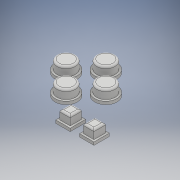
# Autodesk Inventor part: Groboy Buttons
Saved by Autodesk Inventor 2017 SP1 (Build 210196100, 196)
## iProperties
Created: 2017-10-10
Part Number: Groboy Buttons
Material: Generic
Document SubType Name: Modeling
Designer: Groguard
Density: 1 g/cm^3
Appearance: Default
Author: Groguard
Autodesk Inventor part; units mm, degrees
ref_plane "YZ Plane" through (0, 0, 0) normal (1, 0, 0) x (0, 1, 0)
ref_plane "XZ Plane" through (0, 0, 0) normal (0, 1, 0) x (-1, 0, 0)
ref_plane "XY Plane" through (0, 0, 0) normal (0, 0, 1) x (1, 0, 0)
sketch "Sketch1" plane through (0, 0, 0) normal (0, 0, 1) x (1, 0, 0)
  circle A0 centre (22, 46) radius 4.5
  circle A1 centre (12, 36) radius 4.5
  circle A2 centre (22, 26) radius 4.5
  circle A3 centre (32, 36) radius 4.5
  line L0 (37.75, 18) -> (32.5, 18)
  line L1 (32.5, 18) -> (32.5, 12.25)
  line L2 (32.5, 12.25) -> (37.75, 12.25)
  line L3 (37.75, 12.25) -> (37.75, 18)
  line L4 (44.5, 18) -> (49.75, 18)
  line L5 (49.75, 18) -> (49.75, 12.25)
  line L6 (49.75, 12.25) -> (44.5, 12.25)
  line L7 (44.5, 12.25) -> (44.5, 18)
  circle A4 centre (12, 36) radius 5.625
  circle A5 centre (22, 46) radius 5.625
  circle A6 centre (32, 36) radius 5.625
  circle A7 centre (22, 26) radius 5.625
  line L8 (38.75, 19) -> (31.5, 19)
  line L9 (31.5, 19) -> (31.5, 11.25)
  line L10 (31.5, 11.25) -> (38.75, 11.25)
  line L11 (38.75, 11.25) -> (38.75, 19)
  line L12 (50.75, 19) -> (43.5, 19)
  line L13 (43.5, 19) -> (43.5, 11.25)
  line L14 (43.5, 11.25) -> (50.75, 11.25)
  line L15 (50.75, 11.25) -> (50.75, 19)
  point P0 (18.75, 39)
  point P1 (18.75, 32.5)
  dimension "d35" = 11.25
  dimension "d36" = 11.25
  dimension "d37" = 11.25
  dimension "d38" = 11.25
  dimension "d43" = 7.75
  dimension "d44" = 7.75
  dimension "d45" = 7.25
  dimension "d46" = 7.25
  dimension "d47" = 5.75
  dimension "d48" = 5.25
  dimension "d49" = 5.75
  dimension "d50" = 5.25
  constraints: 32 end point, 8 centre point, 8 parallel, 4 perpendicular
  measures "d35" diameter of A4
  measures "d36" diameter of A7
  measures "d37" diameter of A6
  measures "d38" diameter of A5
  measures "d43" distance between parallel lines of L10 L8
  measures "d44" distance between parallel lines of L14 L12
  measures "d45" distance between parallel lines of L11 L9
  measures "d46" distance between parallel lines of L15 L13
  measures "d47" distance between parallel lines of L6 L4
  measures "d48" distance between parallel lines of L7 L5
  measures "d49" distance between parallel lines of L2 L0
  measures "d50" distance between parallel lines of L1 L3
extrude "Extrusion1" add sketch "Sketch1" along normal blind 6 contours A0 | A1 | A2 | A3 | L3 L2 L1 L0 | L4 L5 L6 L7 | A4 | A5 | A6 | A7 | L11 L10 L9 L8 | L15 L14 L13 L12
sketch "Sketch2" plane through (0, 0, 6) normal (0, 0, 1) x (1, 0, 0)
  circle A0 centre (22, 46) radius 4.625
  circle A1 centre (12, 36) radius 4.625
  circle A2 centre (22, 26) radius 4.625
  circle A3 centre (32, 36) radius 4.625
  circle A4 centre (22, 46) radius 5.625
  circle A5 centre (12, 36) radius 5.625
  circle A6 centre (22, 26) radius 5.625
  circle A7 centre (32, 36) radius 5.625
  line L0 (31.5, 19) -> (31.5, 11.25) projected
  line L1 (38.75, 11.25) -> (38.75, 19) projected
  line L2 (31.5, 19) -> (38.75, 19)
  line L3 (38.75, 19) -> (38.75, 11.25)
  line L4 (38.75, 11.25) -> (31.5, 11.25)
  line L5 (31.5, 11.25) -> (31.5, 19)
  line L6 (50.75, 19) -> (43.5, 19) projected
  line L7 (43.5, 11.25) -> (50.75, 11.25) projected
  line L8 (43.5, 19) -> (50.75, 19)
  line L9 (50.75, 19) -> (50.75, 11.25)
  line L10 (50.75, 11.25) -> (43.5, 11.25)
  line L11 (43.5, 11.25) -> (43.5, 19)
  line L12 (37.75, 18) -> (32.5, 18)
  line L13 (32.5, 18) -> (32.5, 12.25)
  line L14 (32.5, 12.25) -> (37.75, 12.25)
  line L15 (37.75, 12.25) -> (37.75, 18)
  line L16 (44.5, 18) -> (49.75, 18)
  line L17 (49.75, 18) -> (49.75, 12.25)
  line L18 (49.75, 12.25) -> (44.5, 12.25)
  line L19 (44.5, 12.25) -> (44.5, 18)
  dimension "d16" = 1
  dimension "d17" = 1
  dimension "d18" = 1
  dimension "d19" = 1
  dimension "d39" = 11.25
  dimension "d40" = 11.25
  dimension "d41" = 11.25
  dimension "d42" = 11.25
  dimension "d51" = 1
  dimension "d52" = 1
  constraints: 32 end point, 8 centre point, 8 parallel, 4 perpendicular, 2 horizontal, 6 other
  measures "d16" radial gap between concentric circles of A0 A4
  measures "d17" radial gap between concentric circles of A1 A5
  measures "d18" radial gap between concentric circles of A2 A6
  measures "d19" radial gap between concentric circles of A3 A7
  measures "d39" diameter of A4
  measures "d40" diameter of A7
  measures "d41" diameter of A6
  measures "d42" diameter of A5
  measures "d51" distance between parallel lines of L2 L12
  measures "d52" distance between parallel lines of L11 L19
extrude "Extrusion2" cut sketch "Sketch2" against normal blind 4.5 contours A4 | A5 | A6 | A7
fillet "Fillet2" radius 1 4 edges at (17.375, 46, 6) (27.375, 36, 6) (17.375, 26, 6) (7.375, 36, 6)
sketch "Sketch5" plane through (0, 0, 6) normal (0, 0, 1) x (1, 0, 0)
  line L0 (31.5, 19) -> (31.5, 11.25) projected
  line L1 (38.75, 11.25) -> (38.75, 19) projected
  line L2 (31.5, 11.25) -> (38.75, 11.25)
  line L3 (38.75, 11.25) -> (38.75, 19)
  line L4 (38.75, 19) -> (31.5, 19)
  line L5 (31.5, 19) -> (31.5, 11.25)
  line L6 (32.5, 18) -> (37.75, 18)
  line L7 (37.75, 18) -> (37.75, 12.25)
  line L8 (37.75, 12.25) -> (32.5, 12.25)
  line L9 (32.5, 12.25) -> (32.5, 18)
  line L10 (43.5, 11.25) -> (50.75, 11.25) projected
  line L11 (50.75, 11.25) -> (50.75, 19) projected
  line L12 (43.5, 11.25) -> (50.75, 11.25)
  line L13 (50.75, 11.25) -> (50.75, 19)
  line L14 (50.75, 19) -> (43.5, 19)
  line L15 (43.5, 19) -> (43.5, 11.25)
  line L16 (44.5, 18) -> (49.75, 18)
  line L17 (49.75, 18) -> (49.75, 12.25)
  line L18 (49.75, 12.25) -> (44.5, 12.25)
  line L19 (44.5, 12.25) -> (44.5, 18)
  point P0 (0, 0)
  point P1 (43.5, 19)
  dimension "d37" = 11.25
  dimension "d58" = 1
  dimension "d60" = 1
  constraints: 32 end point, 8 parallel, 4 perpendicular, 2 horizontal, 6 other
  measures "d58" distance between parallel lines of L4 L6
  measures "d60" distance between parallel lines of L14 L16
extrude "Extrusion5" cut sketch "Sketch5" against normal blind 4.5
fillet "Fillet5" radius 1 8 edges at (32.5, 15.125, 6) (35.125, 12.25, 6) (37.75, 15.125, 6) (35.125, 18, 6) (44.5, 15.125, 6) (47.125, 12.25, 6) (49.75, 15.125, 6) (47.125, 18, 6)
body "Solid1"
